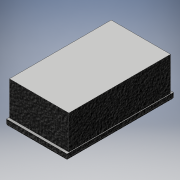
# Autodesk Inventor part: BatteryVoltage
Saved by Autodesk Inventor 2017 (Build 210142000, 142)
## iProperties
Created: 2017-02-10
Part Number: BatteryVoltage
Material: Generic
Document SubType Name: Modeling
Designer: michael
Density: 1 g/cm^3
Appearance: Default
Author: michael
Autodesk Inventor part; units mm, degrees
ref_plane "YZ Plane" through (0, 0, 0) normal (1, 0, 0) x (0, 1, 0)
ref_plane "XZ Plane" through (0, 0, 0) normal (0, 1, 0) x (-1, 0, 0)
ref_plane "XY Plane" through (0, 0, 0) normal (0, 0, 1) x (1, 0, 0)
sketch "Sketch1" plane through (0, 0, 0) normal (0, 1, 0) x (-1, 0, 0)
  line L0 (-12.25, 21) -> (12.25, 21)
  line L1 (12.25, 21) -> (12.25, -21)
  line L2 (12.25, -21) -> (-12.25, -21)
  line L3 (-12.25, -21) -> (-12.25, 21)
  line L4 (-12.25, 21) -> (12.25, -21) construction
  line L5 (12.25, 21) -> (-12.25, -21) construction
  point P0 (0, 0)
  dimension "d0" = 24.5
  dimension "d1" = 42
  constraints: 12 end point, 2 midpoint, 2 parallel, 1 horizontal, 1 perpendicular
  measures "d0" distance of L1.end L2.end
  measures "d1" distance of L0.end L1.end
extrude "Extrusion1" add sketch "Sketch1" along normal blind 14
sketch "Sketch2" plane through (0, 0, 0) normal (0, -1, 0) x (1, 0, 0)
  line L0 (12.5, -22) -> (-12.5, -22)
  line L1 (-12.5, -22) -> (-12.5, 22)
  line L2 (-12.5, 22) -> (12.5, 22)
  line L3 (12.5, 22) -> (12.5, -22)
  line L4 (12.5, -22) -> (-12.5, 22) construction
  line L5 (-12.5, -22) -> (12.5, 22) construction
  point P0 (0, 0)
  dimension "d4" = 25
  dimension "d5" = 44
  constraints: 12 end point, 2 midpoint, 2 parallel, 1 horizontal, 1 perpendicular
  measures "d4" distance of L1.end L2.end
  measures "d5" distance of L0.end L1.end
extrude "Extrusion2" add sketch "Sketch2" along normal blind 2.8
fillet "Fillet1" radius 1.27 4 edges at (0, -2.8, 22) (12.5, -2.8, 0) (0, -2.8, -22) (-12.5, -2.8, 0)
sketch "Sketch3" plane through (0, -2.8, 0) normal (0, -1, 0) x (1, 0, 0)
  line L0 (-11.23, -20.73) -> (-11.23, 20.73) projected
  line L1 (11.23, -20.73) -> (-11.23, -20.73)
  line L2 (-11.23, -20.73) -> (-11.23, 20.73)
  line L3 (-11.23, 20.73) -> (11.23, 20.73)
  line L4 (11.23, 20.73) -> (11.23, -20.73)
  line L5 (11.23, -20.73) -> (-11.23, 20.73) construction
  line L6 (-11.23, -20.73) -> (11.23, 20.73) construction
  point P0 (0, 0)
  constraints: 12 end point, 2 midpoint, 2 parallel, 1 horizontal, 1 perpendicular
extrude "Extrusion3" cut sketch "Sketch3" against normal blind 1.27
body "Solid1"
